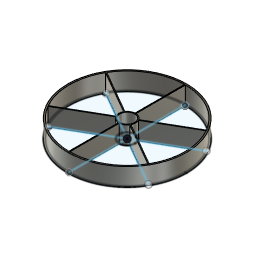
2023_05_22_CD Low PLA wood Storage v3 (Autodesk Fusion 360 design; units mm, degrees)
Autodesk Fusion 360 part; units mm, degrees
sketch "CD Rom Size" plane through (0, 0, 0) normal (0, 0, 1) x (1, 0, 0)
  circle A0 centre (0, 0) radius 7.5
  circle A1 centre (0, 0) radius 7.25
  circle A2 centre (0, 0) radius 60
  circle A3 centre (0, 0) radius 17.5
  dimension "d1" = 15
  dimension "d2" = 14.5
  dimension "d3" = 120
  dimension "d4" = 35
  constraint coincident A0.centre A1.centre
  constraint concentric A0 A1
  constraint concentric A1 A2
  constraint concentric A0 A3
  measures "d1" diameter of A0
  measures "d2" diameter of A1
  measures "d3" diameter of A2
  measures "d4" diameter of A3
extrude "Extrude1" add sketch "CD Rom Size" along normal blind 1.2 contours A2 makes body 1
extrude "Extrude2" add sketch "CD Rom Size" along normal blind 1.19 contours A3 bodies 1
copy_body "CopyPasteBodies1" bodies 1 makes body 2
move_body "Move1" bodies 2 to x (1, 0, 0) y (0, 1, 0) z (0, 0, 1) at (-170, 0, 0)
sketch "Sketch2" plane through (0, 0, 0) normal (0, 0, 1) x (1, 0, 0)
  circle A0 centre (0, 0) radius 60
  circle A1 centre (0, 0) radius 58.5
  line L0 (0.3951, -58.5) -> (0.3951, 58.5)
  arc A2 (0.3951, 58.5) -> (-0.5049, 58.5) centre (-0.0549, 58.5) ccw
  line L1 (-0.5049, 58.5) -> (-0.5049, -58.5)
  arc A3 (-0.5049, -58.5) -> (0.3951, -58.5) centre (-0.0549, -58.5) ccw
  line L2 (-0.0549, -58.5) -> (-0.0549, 58.5) construction
  line L3 (-50.41, -29.6873) -> (50.9149, 28.8127)
  arc A4 (50.9149, 28.8127) -> (50.4649, 29.5921) centre (50.6899, 29.2024) ccw
  arc A5 (-50.86, -28.9079) -> (-50.41, -29.6873) centre (-50.635, -29.2976) ccw
  line L4 (50.4649, 29.5921) -> (-50.86, -28.9079)
  line L5 (50.9149, -28.8127) -> (-50.41, 29.6873)
  arc A6 (-50.41, 29.6873) -> (-50.86, 28.9079) centre (-50.635, 29.2976) ccw
  arc A7 (50.4649, -29.5921) -> (50.9149, -28.8127) centre (50.6899, -29.2024) ccw
  line L6 (-50.86, 28.9079) -> (50.4649, -29.5921)
  dimension "d21" = 117
  dimension "d22" = 120
  dimension "d23" = 0.9
  dimension "d25" = 360
  constraint coincident A0.centre A1.centre
  constraint tangent L0 A2
  constraint tangent A2 L1
  constraint parallel L0 L1
  constraint tangent L1 A3
  constraint tangent L0 A3
  constraint coincident A1 A2.centre
  constraint vertical L2
  constraint coincident A1 A3.centre
  measures "d21" diameter of A1
  measures "d22" diameter of A0
  measures "d23" diameter of A2
extrude "Extrude3" add sketch "Sketch2" along normal blind 18 separate body contours A0 | A1 A4 | A1 A2 L1 | A1 A6 | A1 A7 | A1 A5 | A1 L1 A3 makes body 3
sketch "Sketch3" plane through (0, 0, 0) normal (0, 0, 1) x (1, 0, 0)
  circle A0 centre (0, 0) radius 7.5
  circle A1 centre (0, 0) radius 8.5
  dimension "d14" = 15
  dimension "d15" = 17
  constraint coincident A0.centre A1.centre
  measures "d14" diameter of A0
  measures "d15" diameter of A1
extrude "Extrude4" add sketch "Sketch3" sketch "Sketch2" along normal blind 18 contours A0 of sketch 2 contours A1 L0 L3 L4 L5 | A1 L0 L1 L4 L5 | A1 L0 L3 L5 L6 | A1 L1 L4 L5 L6 | A1 L0 L1 L3 L6 | A1 L1 L3 L4 L6 bodies 3
extrude "Extrude5" add sketch "Sketch3" along normal blind 18 bodies 3
extrude "Extrude6" cut sketch "Sketch3" along normal blind 18 contours A0 bodies 3
sketch "Sketch4" plane through (0, 0, 0) normal (0, 0, 1) x (1, 0, 0)
  circle A0 centre (0, 58.5) radius 2.0493
  circle A1 centre (0, 58.5) radius 3.1171
  line L0 (0, 58.5) -> (-3.1171, 58.5)
  line L1 (0, 58.5) -> (3.1171, 58.5)
  constraint concentric A0 A1
  constraint coincident A0.centre A1.centre
  constraint coincident A1 L0.end
  constraint horizontal L0
  constraint coincident A1 L1.end
  constraint parallel L0 L1
extrude "Extrude7" add sketch "Sketch4" along normal blind 0.6 separate body contours A0 A1 L0 L1 picked at (2.7419, 58.2433) makes body 4
pattern_circular "C-Pattern1" count 6 over 360 about axis through (0, 0, 1.75) along (0, 0, 1) of bodies 4 makes body 5 at (-49.1536, 31.5538, 0) makes body 6 at (-51.8112, -26.7471, 0) makes body 7 at (-2.7419, -58.2433, 0) makes body 8 at (49.0692, -31.4962, 0) makes body 9 at (51.9032, 26.7914, 0)
combine "Combine1" operation add target body 3 tool bodies 4 9 5 6 7 8
hidden bodies 1 2
equation "d11 = WoodSize"
equation "WoodSize = 18 mm"
equation "d16 = WoodSize"
equation "d18 = WoodSize"
equation "d26 = WoodSize"
named bodies: "LowCutPla"
